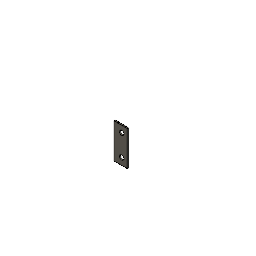
Printed_Mount_Spacer (Autodesk Fusion 360 design; units mm, degrees)
Autodesk Fusion 360 part; units mm, degrees
sketch "Sketch1" plane through (0, 0, 416.85) normal (0, 0, -1) x (1, 0, 0)
  circle A0 centre (235.386, 254.9414) radius 1.6
  circle A1 centre (235.386, 270.828) radius 1.6
  line L0 (239.6286, 249.9414) -> (239.6286, 275.9414)
  line L1 (239.6286, 275.9414) -> (229.6286, 275.9414)
  line L2 (229.6286, 275.9414) -> (229.6286, 249.9414)
  line L3 (229.6286, 249.9414) -> (239.6286, 249.9414)
extrude "Extrude1" add sketch "Sketch1" along normal blind 1
